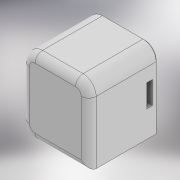
# Autodesk Inventor part: Cap
Saved by Autodesk Inventor 2020 (Build 240168000, 168)
## iProperties
Created: 2022-04-06
Part Number: Cap
Material: 일반
Document SubType Name: Modeling
Designer: Knowblesse
Density: 1 g/cm^3
Appearance: 기본값
Author: Knowblesse
## iProperties of the stored document _3D 인쇄.ipt
Created: 2022-04-06
Part Number: _3D 인쇄
Material: 일반
Document SubType Name: Modeling
Designer: Knowblesse
Density: 1 g/cm^3
Appearance: 기본값
Author: Knowblesse
Autodesk Inventor part; units mm, degrees
ref_plane "YZ Plane" through (0, 0, 0) normal (1, 0, 0) x (0, 1, 0)
ref_plane "XZ Plane" through (0, 0, 0) normal (0, 1, 0) x (-1, 0, 0)
ref_plane "XY Plane" through (0, 0, 0) normal (0, 0, 1) x (1, 0, 0)
sketch "스케치1" plane through (0, 0, 0) normal (0, 0, 1) x (1, 0, 0)
  line L0 (-5.4, -8.6) -> (7.4, -8.6)
  line L1 (7.4, -8.6) -> (7.4, 6.6)
  line L2 (5.4, 8.6) -> (-5.4, 8.6)
  line L3 (-7.4, 6.6) -> (-7.4, -6.6)
  line L4 (-7.4, -8.6) -> (7.4, 8.6) construction
  line L5 (7.4, -8.6) -> (-7.4, 8.6) construction
  arc A0 (-5.4, 8.6) -> (-7.4, 6.6) centre (-5.4, 6.6) ccw
  arc A1 (7.4, 6.6) -> (5.4, 8.6) centre (5.4, 6.6) ccw
  arc A2 (-7.4, -6.6) -> (-5.4, -8.6) centre (-5.4, -6.6) ccw
  line L6 (-5.4, 10.1) -> (5.4, 10.1)
  arc A3 (8.9, 6.6) -> (5.4, 10.1) centre (5.4, 6.6) ccw
  line L7 (8.9, 6.6) -> (8.9, -10.1)
  line L8 (8.9, -10.1) -> (-5.4, -10.1)
  arc A4 (-8.9, -6.6) -> (-5.4, -10.1) centre (-5.4, -6.6) ccw
  line L9 (-8.9, -6.6) -> (-8.9, 6.6)
  arc A5 (-5.4, 10.1) -> (-8.9, 6.6) centre (-5.4, 6.6) ccw
  point P0 (0, 0)
  dimension "d0" = 17.2
  dimension "d1" = 14.8
  dimension "d2" = 2
  dimension "d3" = 1.5
  constraints: 20 end point, 12 point on circle, 6 centre point, 6 point on line, 6 tangent, 4 parallel, 2 equal radius, 2 midpoint, 2 perpendicular, 1 horizontal, 6 other
  measures "d0" distance of L0.end L4.end
  measures "d1" distance of L4.end L5.end
  measures "d2" radius of A0
  measures "d3" distance between parallel lines of L2 L6
extrude "돌출1" add sketch "스케치1" along normal blind 17
sketch "스케치2" plane through (0, 0, 17) normal (0, 0, 1) x (1, 0, 0)
  line L0 (-5.4, -10.1) -> (8.9, -10.1) projected
  line L1 (8.9, -10.1) -> (8.9, 6.6) projected
  arc A0 (8.9, 6.6) -> (5.4, 10.1) centre (5.4, 6.6) ccw projected
  line L2 (5.4, 10.1) -> (-5.4, 10.1) projected
  arc A1 (-5.4, 10.1) -> (-8.9, 6.6) centre (-5.4, 6.6) ccw projected
  line L3 (-8.9, 6.6) -> (-8.9, -6.6) projected
  arc A2 (-8.9, -6.6) -> (-5.4, -10.1) centre (-5.4, -6.6) ccw projected
  point P0 (0, 0)
extrude "돌출2" add sketch "스케치2" along normal blind 1.5
sketch "스케치3" plane through (-8.9, -6.6, 0) normal (-1, 0, 0) x (0, 0, 1)
  line L0 (0, 13.2) -> (0, 0) projected
  line L1 (3, 3.6) -> (1.5, 3.6)
  line L2 (1.5, 3.6) -> (1.5, 9.6)
  line L3 (1.5, 9.6) -> (3, 9.6)
  line L4 (3, 9.6) -> (3, 3.6)
  point P0 (0, 6.6)
  point P1 (0, 6.6)
  point P2 (1.5, 6.6)
  dimension "d8" = 6
  dimension "d9" = 1.5
  dimension "d10" = 1.5
  constraints: 8 end point, 2 midpoint, 2 parallel, 1 horizontal, 1 horizontal alignment, 1 perpendicular
  measures "d8" distance of L1.end L2.end
  measures "d9" distance of L2.end L3.end
  measures "d10" distance between parallel lines of L2 L0
extrude "돌출3" cut sketch "스케치3" against normal through all
fillet "모깎기1" radius 2 7 edges at (-7.8749, -9.0749, 18.5) (1.75, -10.1, 18.5) (-7.8749, 9.0749, 18.5) (0, 10.1, 18.5) (7.8749, 9.0749, 18.5) (8.9, -1.75, 18.5) (-8.9, 0, 18.5)
chamfer "모따기1" distance 0.5 angle 45 7 edges at (1.75, -10.1, 0) (-7.8749, -9.0749, 0) (-8.9, 0, 0) (-7.8749, 9.0749, 0) (0, 10.1, 0) (7.8749, 9.0749, 0) (8.9, -1.75, 0)
sketch "스케치4" plane through (-5.4, -10.1, 16.5) normal (0, -1, 0) x (1, 0, 0)
  line L0 (1.75, -14.5) -> (3.25, -14.5)
  line L1 (3.25, -14.5) -> (3.25, -16.5)
  line L2 (3.25, -16.5) -> (1.75, -16.5)
  line L3 (1.75, -16.5) -> (1.75, -14.5)
  line L4 (-3.5, -16) -> (-3.5, 0) projected
  line L5 (0, -16.5) -> (13.8, -16.5) projected
  point P0 (5.4, -16.5)
  point P1 (2.5, -14.5)
  point P2 (2.5, -14.5)
  dimension "d17" = 1.5
  dimension "d18" = 2
  dimension "d19" = 6
  constraints: 8 end point, 2 parallel, 1 coincident, 1 collinear, 1 horizontal, 1 midpoint, 1 perpendicular
  measures "d17" distance of L1.end L2.end
  measures "d18" distance of L0.end L1.end
  measures "d19" distance from line of L4 point (2.5, -14.5)
extrude "돌출4" cut sketch "스케치4" against normal up to surface (1.5 mm away)
